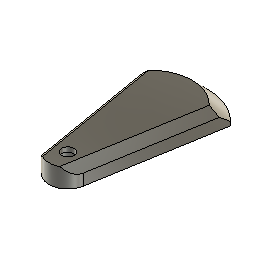
Compact_Robot_Body66 v1 (Autodesk Fusion 360 design; units mm, degrees)
Autodesk Fusion 360 part; units mm, degrees
sketch "Esboço1" plane through (0, 0, 0) normal (0, 0, 1) x (1, 0, 0)
  line L0 (0, 5) -> (0, 6.96) construction
  line L1 (-4.9294, -0.8373) -> (-10.6041, 32.5691)
  line L2 (4.9294, -0.8373) -> (10.6041, 32.5691)
  arc A0 (10.6041, 32.5691) -> (-10.6041, 32.5691) centre (0, 21.96) ccw
  arc A1 (-4.9294, -0.8373) -> (4.9294, -0.8373) centre (0, 0) ccw
  circle A2 centre (0, 0) radius 3
  circle A3 centre (0, 0) radius 1.65
  dimension "d1" = 10
  dimension "d2" = 21.96
  dimension "d3" = 30
  dimension "d4" = 33.885
  dimension "d5" = 33.885
  dimension "d8" = 6
  dimension "d9" = 3.3
  constraint coincident A1.centre A2.centre
  constraint vertical L0
  constraint tangent L1 A1
  constraint tangent L2 A1
  constraint concentric A1 A3
  measures "d1" diameter of A1
  measures "d2" distance of A1.centre A0.centre
  measures "d3" diameter of A0
  measures "d4" distance of L1.start L1.end
  measures "d5" distance of L2.start L2.end
  measures "d8" diameter of A2
  measures "d9" diameter of A3
extrude "Extrusão1" add sketch "Esboço1" along normal blind 5 contours L1 L2 A0 A1 | A2 | A3
extrude "Extrusão2" cut sketch "Esboço1" along normal blind 28 contours A3
extrude "Extrusão3" cut sketch "Esboço1" along normal blind 3.75 contours A2
chamfer "Chanfro1" distance 2 angle 45 2 edges at (7.7667, 15.8659, 5) (-7.7667, 15.8659, 5)
chamfer "Chanfro2" distance 4 angle 45 1 edges at (0, 36.96, 5)
